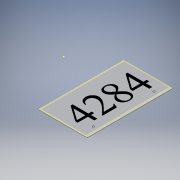
# Autodesk Inventor part: Plexiglass number plate 2
Saved by Autodesk Inventor 2019 (Build 230136000, 136)
## iProperties
Created: 2019-02-04
Part Number: Plexiglass number plate 2
Material: Generic
Document SubType Name: Modeling
Designer: mrhftc
Density: 1 g/cm^3
Appearance: Default
Author: mrhftc
Autodesk Inventor part; units mm, degrees
ref_plane "YZ Plane" through (0, 0, 0) normal (1, 0, 0) x (0, 1, 0)
ref_plane "XZ Plane" through (0, 0, 0) normal (0, 1, 0) x (-1, 0, 0)
ref_plane "XY Plane" through (0, 0, 0) normal (0, 0, 1) x (1, 0, 0)
sketch "Sketch1" plane through (0, 0, 0) normal (0, 1, 0) x (-1, 0, 0)
  line L0 (-68.8755, 120.8229) -> (-170.4755, 120.8229)
  line L1 (-170.4755, 120.8229) -> (-170.4755, -56.9771)
  line L2 (-170.4755, -56.9771) -> (-68.8755, -56.9771)
  line L3 (-68.8755, -56.9771) -> (-68.8755, 120.8229)
  circle A0 centre (-157.7755, 95.4229) radius 2.1
  circle A1 centre (-157.7755, -31.5771) radius 2.1
  point P0 (0, 0)
  dimension "d0" = 101.6
  dimension "d1" = 177.8
  dimension "d15" = 127
  dimension "d16" = 12.7
  dimension "d17" = 25.4
  dimension "d18" = 12.7
  constraints: 8 end point, 2 centre point, 2 parallel, 1 horizontal, 1 perpendicular
  measures "d0" distance between parallel lines of L1 L3
  measures "d1" distance between parallel lines of L2 L0
  measures "d15" distance of A0.centre A1.centre
  measures "d16" distance from line of L1 A1.centre
  measures "d17" distance from line of L0 A0.centre
  measures "d18" distance from line of L1 A0.centre
extrude "Extrusion2" add sketch "Sketch1" along normal blind 1.27
sketch "Sketch2" plane through (0, 1.27, 0) normal (0, 1, 0) x (1, 0, 0)
  line L0 (68.8755, -120.8229) -> (170.4755, -120.8229) construction
  line L1 (170.4755, -120.8229) -> (170.4755, 56.9771) construction
  line L2 (170.4755, 56.9771) -> (68.8755, 56.9771) construction
  line L3 (68.8755, 56.9771) -> (68.8755, -120.8229) construction
  line L4 (71.2877, -118.5262) -> (71.2877, 55.6852) construction
  line L5 (71.2877, 55.6852) -> (165.8932, 55.6852) construction
  line L6 (165.8932, 55.6852) -> (165.8932, -118.5262) construction
  line L7 (165.8932, -118.5262) -> (71.2877, -118.5262) construction
  point P0 (0, 0)
  constraints: 2 other
body "Solid2"
